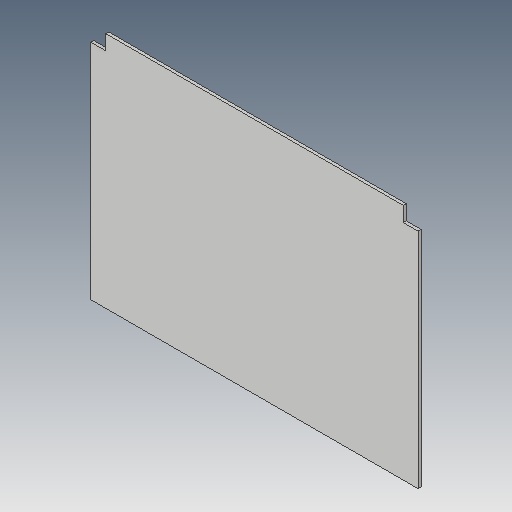
# Autodesk Inventor part: 防水p3
Saved by Autodesk Inventor 2020.3 (Build 243373000, 373)
## iProperties
Part Number: 防水p3
Material: 一般
Document SubType Name: Modeling
Designer: highs
Density: 1 g/cm^3
Appearance: 既定
Author: highs
Autodesk Inventor part; units mm, degrees
ref_plane "YZ Plane" through (0, 0, 0) normal (1, 0, 0) x (0, 1, 0)
ref_plane "XZ Plane" through (0, 0, 0) normal (0, 1, 0) x (-1, 0, 0)
ref_plane "XY Plane" through (0, 0, 0) normal (0, 0, 1) x (1, 0, 0)
sketch "スケッチ1" plane through (0, 0, 0) normal (0, 0, 1) x (1, 0, 0)
  line L0 (0, 0) -> (440, 0)
  line L1 (440, 0) -> (440, 320)
  line L2 (440, 320) -> (0, 320)
  line L3 (0, 320) -> (0, 0)
  dimension "d0" = 440
  dimension "d1" = 320
  constraints: 8 end point, 2 parallel, 1 horizontal, 1 perpendicular
  measures "d0" distance of L0.start L0.end
  measures "d1" distance of L2.end L0.start
extrude "押し出し1" add sketch "スケッチ1" along normal blind 4
sketch "スケッチ2" plane through (0, 0, 4) normal (0, 0, 1) x (1, 0, 0)
  line L0 (440, 320) -> (0, 320) projected
  line L1 (0, 320) -> (20, 320)
  line L2 (20, 320) -> (20, 300)
  line L3 (20, 300) -> (0, 300)
  line L4 (0, 300) -> (0, 320)
  line L5 (440, 320) -> (420, 320)
  line L6 (420, 320) -> (420, 300)
  line L7 (420, 300) -> (440, 300)
  line L8 (440, 300) -> (440, 320)
  point P0 (0, 0)
  dimension "d4" = 20
  constraints: 16 end point, 4 parallel, 2 equal length, 2 horizontal, 2 perpendicular, 1 point on line
  measures "d4" distance of L2.end L3.end
extrude "押し出し2" cut sketch "スケッチ2" against normal blind 10
